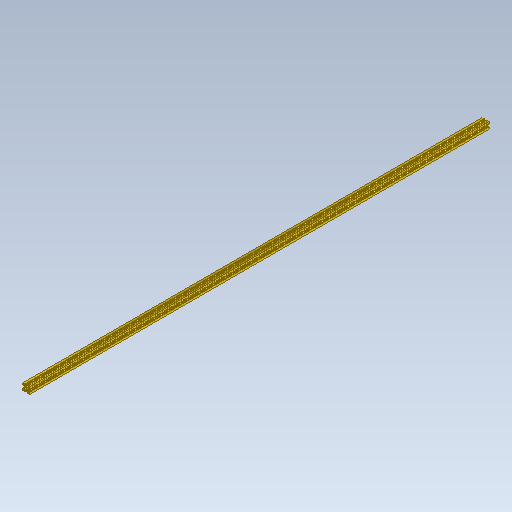
# Autodesk Inventor part: Perfil 30×30 2 rasgos opostos_AST03003002O
Saved by Autodesk Inventor 2025.2 (Build 292293000, 293)
## iProperties
Created: 2025-04-06
Part Number: Perfil 30×30 2 rasgos opostos_AST03003002O
Material: Ouro
Document SubType Name: Modeling
Designer: Gustavo Sousa
Density: 19.3 g/cm^3
Appearance: Metal quente 2400F
Author: Gustavo Sousa
Autodesk Inventor part; units mm, degrees
ref_plane "YZ Plane" through (0, 0, 0) normal (1, 0, 0) x (0, 1, 0)
ref_plane "XZ Plane" through (0, 0, 0) normal (0, 1, 0) x (-1, 0, 0)
ref_plane "XY Plane" through (0, 0, 0) normal (0, 0, 1) x (1, 0, 0)
sketch "Esboço1" plane through (0, 0, 0) normal (0, 0, 1) x (1, 0, 0)
  circle A0 centre (0, 0) radius 5 construction
  line L0 (-15, 15) -> (15, 15) construction
  arc A1 (0, 5) -> (-5, 0) centre (0, 0) ccw
  line L1 (-3.5355, 3.5355) -> (0, 0) construction
  line L2 (-3.5355, 3.5355) -> (-15, 15) construction
  line L3 (-7, 7) -> (7, 7) construction
  line L4 (-15, 15) -> (-15, -15) construction
  line L5 (-7, 7) -> (-7, -7) construction
  line L6 (-15, 4.1) -> (-15, -4.1)
  line L7 (-15, 4.1) -> (-12.8, 4.1) construction
  line L8 (-12.8, 4.1) -> (-12.8, 8.15) construction
  line L9 (-9.7056, 8.15) -> (-7, 5.4444) construction
  line L10 (-12.8, 8.15) -> (-9.7056, 8.15) construction
  line L11 (-7, 5.4444) -> (-7, 0) construction
  line L12 (-15, 4.1) -> (-14.5, 4.1) construction
  line L13 (-14.5, 4.1) -> (-14.5, 4.6)
  line L14 (-14.5, 4.6) -> (-15, 4.6)
  line L15 (-15, 4.6) -> (-15, 4.1) construction
  line L16 (-14.5, 4.1) -> (-12.8, 4.1)
  line L17 (-15, 14.5) -> (-15, 4.6)
  circle A2 centre (-11.5, 11.5) radius 2.25
  line L18 (-11.5, 11.5) -> (-11.5, 13.75) construction
  circle A3 centre (-3.5355, 3.5355) radius 1.1 construction
  arc A4 (-2.6769, 4.2231) -> (-4.2231, 2.6769) centre (-3.5355, 3.5355) ccw
  line L19 (-7, 0) -> (-5, 0)
  arc A5 (-12.3, 8.15) -> (-12.8, 7.65) centre (-12.3, 7.65) ccw
  arc A6 (-9.5592, 8.0036) -> (-9.9127, 8.15) centre (-9.9127, 7.65) ccw
  arc A7 (-7, 5.2373) -> (-7.1464, 5.5908) centre (-7.5, 5.2373) ccw
  line L20 (-12.8, 7.65) -> (-12.8, 4.1)
  line L21 (-12.3, 8.15) -> (-9.9127, 8.15)
  line L22 (-9.5592, 8.0036) -> (-7.1464, 5.5908)
  line L23 (-7, 5.2373) -> (-7, 0)
  line L24 (-14.8536, 14.8536) -> (-13.091, 13.091)
  line L25 (-9.909, 9.909) -> (-4.3134, 4.3134)
  arc A8 (-14.5, 15) -> (-15, 14.5) centre (-14.5, 14.5) ccw construction
  arc A9 (-14.8536, 14.8536) -> (-15, 14.5) centre (-14.5, 14.5) ccw
  point P0 (-15, 0)
  point P1 (-15, 0)
  point P2 (-12.3, 8.15)
  point P3 (0, 7)
  dimension "d0" = 10
  dimension "d1" = 15
  dimension "d2" = 30
  dimension "d5" = 8.2
  dimension "espessura" = 2.2
  dimension "d7" = 1.1
  dimension "quadrado" = 0.5
  dimension "d10" = 4.5
  dimension "d13" = 1.1
  dimension "d14" = 11.5
  dimension "d21" = 2.2
  dimension "d41" = 0.5
  dimension "d42" = 2
  dimension "d44" = 8
  constraints: 52 end point, 26 point on circle, 13 point on line, 10 centre point, 10 tangent, 6 perpendicular, 5 collinear, 5 equal radius, 5 horizontal, 4 coincident, 4 midpoint, 4 vertical, 3 horizontal alignment, 3 parallel, 2 vertical alignment
  measures "d0" diameter of A0
  measures "d1" distance from line of point (0, 0) L0
  measures "d2" distance of L0.start L0.end
  measures "d5" distance of L6.start L6.end
  measures "espessura" distance between parallel lines of L4 L8
  measures "d7" distance between parallel lines of L2 L9
  measures "quadrado" distance of L13.end L14.end
  measures "d10" diameter of A2
  measures "d13" distance edge to line of A2 L10
  measures "d14" horizontal distance of point (0, 0) L18.start
  measures "d21" diameter of A3
  measures "d41" radius of A8
  measures "d42" distance from line of A0.start L3
  measures "d44" distance between parallel lines of L5 L4
extrude "Extrusão7" add sketch "Esboço1" along normal mid plane 2000 contours A1 L19 L23 A7 L22 A6 L21 A5 L20 L16 L13 L14 L17 A9 L24 A2 L25 A4
mirror "Espelhar15" about plane through (0, 0, 0) normal (0, 1, 0) of "Extrusão7"
mirror "Espelhar16" about plane through (0, 0, 0) normal (1, 0, 0) of "Extrusão7", "Espelhar15"
mirror "Espelhar17" about plane through (-4.3134, -4.3134, 0) normal (0.7071068, -0.7071068, 0) of "Extrusão7", "Espelhar15"
mirror "Espelhar18" about plane through (0, 0, 0) normal (0, 1, 0) of "Extrusão7", "Espelhar15", "Espelhar17"
equation "\"d13\" = 0.5 * espessura"
